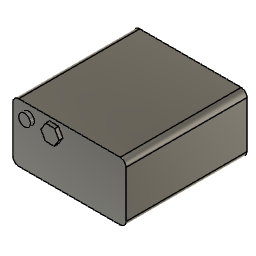
Bloc pile 12V v1 (Autodesk Fusion 360 design; units mm, degrees)
Autodesk Fusion 360 part; units mm, degrees
sketch "Esquisse1" plane through (0, 0, 0) normal (0, 0, 1) x (1, 0, 0)
  line L0 (0, 0) -> (58, 0)
  line L1 (58, 0) -> (58, 62)
  line L2 (58, 62) -> (0, 62)
  line L3 (0, 62) -> (0, 0)
  dimension "d1" = 58
  dimension "d2" = 62
  constraint horizontal L0
  constraint vertical L1
  constraint horizontal L2
  constraint vertical L3
  constraint coincident L0.start L3.end
  measures "d1" distance of L0.start L0.end
  measures "d2" distance of L0.start L2.end
extrude "Extrusion1" add sketch "Esquisse1" along normal blind 30
fillet "Congé1" radius 3 4 edges at (58, 31, 30) (58, 31, 0) (0, 31, 30) (0, 31, 0)
sketch "Esquisse2" plane through (0, 0, 0) normal (0, -1, 0) x (1, 0, 0)
  arc A0 (0, 3) -> (3, 0) centre (3, 3) ccw
  line L0 (3, 0) -> (55, 0)
  arc A1 (55, 0) -> (58, 3) centre (55, 3) ccw
  line L1 (58, 3) -> (58, 27)
  arc A2 (58, 27) -> (55, 30) centre (55, 27) ccw
  line L2 (55, 30) -> (3, 30)
  arc A3 (3, 30) -> (0, 27) centre (3, 27) ccw
  line L3 (0, 27) -> (0, 3)
  circle A4 centre (8, 24) radius 3
  dimension "d7" = 6
  dimension "d8" = 6
  dimension "d9" = 8
  measures "d7" diameter of A4
  measures "d8" distance of L2 A4.centre
  measures "d9" distance of L3 A4.centre
sketch "Esquisse3" plane through (0, 0, 0) normal (0, -1, 0) x (1, 0, 0)
  line L0 (18.832, 28.0784) -> (16.384, 24.1616)
  line L1 (16.384, 24.1616) -> (18.552, 20.0833)
  line L2 (18.552, 20.0833) -> (23.168, 19.9216)
  line L3 (23.168, 19.9216) -> (25.616, 23.8384)
  line L4 (25.616, 23.8384) -> (23.448, 27.9167)
  line L5 (23.448, 27.9167) -> (18.832, 28.0784)
  line L6 (55, 30) -> (3, 30)
  line L7 (0, 27) -> (0, 3)
  point P0 (21, 24)
  dimension "d10" = 8
  dimension "d11" = 6
  dimension "d12" = 21
  measures "d10" distance of L2 L5
  measures "d11" distance of P0 L6
  measures "d12" distance of P0 L7
extrude "Extrusion2" add sketch "Esquisse2" sketch "Esquisse3" along normal blind 2 contours A4 of sketch 2
